Autodesk Fusion 360 part; units mm, degrees
note: some values were not read from the file. Set by a fixed rule: which sketch regions a step uses.
(part 2 of 2)
sketch "スケッチ2" plane through (0, 0, -13.6) normal (0, 0, -1) x (1, 0, 0)
  line L0 (102.5, -6.3) -> (102.5, 113.7)
  line L1 (-7.5, 113.7) -> (-7.5, -6.3)
  line L2 (-7.5, -6.3) -> (102.5, -6.3)
  line L3 (102.5, -6.3) -> (-7.5, -6.3)
  line L4 (102.5, -6.3) -> (88.1851, -6.3)
  line L5 (6.8149, -6.3) -> (-7.5, -6.3)
  arc A0 (79.5945, -2.1704) -> (15.4055, -2.1704) centre (47.5, -27.8382) ccw
  arc A1 (79.5945, -2.1704) -> (88.1851, -6.3) centre (88.1851, 4.7) ccw
  arc A2 (6.8149, -6.3) -> (15.4055, -2.1704) centre (6.8149, 4.7) ccw
  dimension "d131" = 11
  dimension "d132" = 11
  constraint coincident L0.start L2.end
  constraint coincident L1.end L2.start
  constraint tangent L4 A1
  constraint tangent A0 A1
  constraint tangent L5 A2
  constraint tangent A0 A2
  measures "d131" radius of A1
  measures "d132" radius of A2
sketch "スケッチ3" plane through (-7.5, 0, 0) normal (-1, 0, 0) x (0, -1, 0)
  line L0 (-6.3, 0) -> (-6.3, -13.6)
  line L1 (-6.3, -13.6) -> (113.7, -13.6)
  line L2 (113.7, -13.6) -> (113.7, 0)
  line L3 (113.7, -13.6) -> (-6.3, -13.6)
  line L4 (-6.3, -13.6) -> (-6.3, -26.6)
  line L5 (62.6427, -19.1312) -> (113.7, -13.6)
  line L6 (-6.3, -13.6) -> (-4.908, -26.4492)
  line L7 (113.7, -13.6) -> (112.2266, 0.0005)
  line L8 (112.2266, 0.0005) -> (113.7, 0)
  line L9 (113.7, -13.6) -> (113.7, 0)
  line L10 (113.7, 0) -> (103.9, 0)
  line L11 (103.9, 0) -> (95.0048, 0.2938)
  line L12 (103.9, 0) -> (113.7, -13.6)
  line L13 (113.7, 0) -> (113.6982, -5)
  line L14 (113.6982, -5) -> (113.6982, -8)
  line L15 (95.0048, 0.2938) -> (94.7516, -7.3743)
  line L16 (103.9, 0) -> (103.6468, -7.668)
  line L17 (113.6982, -5) -> (94.8506, -4.3775)
  line L18 (113.6982, -8) -> (94.7516, -7.3743)
  line L19 (95.0048, 0.2938) -> (107.3519, -4.7904)
  line L20 (-4.908, -26.4492) -> (113.7, -13.6)
  line L21 (15.8428, -24.2012) -> (-4.908, -26.4492)
  line L22 (24.744, -23.2369) -> (-4.908, -26.4492)
  line L23 (9.918, -24.8431) -> (9.918, -13.6)
  arc A0 (58.2791, -18.1695) -> (19.8991, -22.3273) centre (41.8256, -45.5076) ccw
  arc A1 (15.8428, -24.2012) -> (19.8991, -22.3273) centre (15.0888, -17.2419) ccw
  arc A2 (58.2791, -18.1695) -> (62.6427, -19.1312) centre (61.8888, -12.1719) ccw
  line L24 (113.7, 0) -> (125.4418, 0)
  line L25 (125.4418, 0) -> (125.4418, -18.6195)
  line L26 (125.4418, -18.6195) -> (113.7, -18.6195)
  line L27 (113.7, -18.6195) -> (113.7, 0)
  line L28 (-4.908, -26.4492) -> (-6.3, -26.6)
  line L29 (-6.3, -13.6) -> (128.5492, -13.6)
  line L30 (128.5492, -13.6) -> (128.5492, -27.0128)
  line L31 (128.5492, -27.0128) -> (-6.3, -27.0128)
  line L32 (-6.3, -27.0128) -> (-6.3, -13.6)
  line L33 (113.7, 0) -> (-6.3, 0)
  dimension "d133" = 13
  dimension "d146" = 9.8
  dimension "d147" = 8.9
  dimension "d148" = 5
  dimension "d149" = 3
  dimension "d160" = 7
  dimension "d161" = 7
  constraint coincident L1.end L2.start
  constraint coincident L0.end L1.start
  constraint perpendicular L3 L4
  constraint coincident L5 L6.end
  constraint perpendicular L5 L6
  constraint perpendicular L5 L7
  constraint coincident L2.end L8.end
  constraint perpendicular L9 L10
  constraint perpendicular L8 L13
  constraint parallel L9 L14
  constraint perpendicular L11 L15
  constraint perpendicular L11 L16
  constraint coincident L15 L17.end
  constraint perpendicular L15 L17
  constraint perpendicular L15 L18
  constraint coincident L18 L16.end
  constraint coincident L12 L19.end
  constraint coincident L17 L19.end
  constraint midpoint L22 L23.start
  constraint coincident L3 L23.end
  constraint perpendicular L3 L23
  constraint tangent L23 A0
  constraint tangent L3 A0
  constraint coincident L21 L22.start
  constraint tangent A0 A1
  constraint tangent L21 A1
  constraint tangent A0 A2
  constraint tangent L5 A2
  constraint horizontal L24
  constraint vertical L25
  constraint horizontal L26
  constraint vertical L27
  constraint parallel L22 L28
  constraint horizontal L29
  constraint vertical L30
  constraint horizontal L31
  constraint vertical L32
  measures "d133" distance of L0.end L4.end
  measures "d146" distance of L2.end L10.end
  measures "d147" distance of L10.end L11.end
  measures "d148" distance of L2.end L13.end
  measures "d149" distance of L13.end L14.end
  measures "d160" radius of A1
  measures "d161" radius of A2
extrude "押し出し9" add sketch "スケッチ3" against normal blind 110 contours L1 L3 L6 L20 L21 L22 L23 L29 | L1 L3 L20 L21 L22 L23 A0 A1 L29 | L1 L3 L5 L20 A0 A2 L29 | L20 L22 A0 A1 A2
extrude "押し出し10" cut 2 faces at (11.85, -19.9223, 0) (11.85, -19.9223, 0) along direction (0, 0, -1) blind 0.1
extrude "押し出し11" cut sketch "スケッチ2" along normal blind 16 and the other way blind 2
sketch "スケッチ8" plane through (0, 6.3, 0) normal (0, 1, 0) x (-1, 0, 0)
  line L0 (-6.8149, -11.7) -> (-6.8149, -13.6)
  line L1 (-6.8149, -13.6) -> (7.5, -13.6)
  line L2 (7.5, -13.6) -> (7.5, -0.1)
  line L3 (7.5, -0.1) -> (-102.5, -0.1)
  line L4 (-102.5, -0.1) -> (-102.5, -13.6)
  line L5 (-102.5, -13.6) -> (-88.1851, -13.6)
  line L6 (-88.1851, -13.6) -> (-88.1851, -11.7)
  line L7 (-88.1851, -11.7) -> (-97.7, -11.7)
  line L8 (-97.7, -11.7) -> (-97.7, -10.5)
  line L9 (-97.7, -10.5) -> (-87.7, -10.5)
  line L10 (-87.7, -10.5) -> (-87.7, -8.7)
  line L11 (-87.7, -8.7) -> (-97.7, -8.7)
  line L12 (-97.7, -8.7) -> (-97.7, -2.9)
  line L13 (-97.7, -2.9) -> (2.7, -2.9)
  line L14 (2.7, -2.9) -> (2.7, -8.7)
  line L15 (2.7, -8.7) -> (-7.3, -8.7)
  line L16 (-7.3, -8.7) -> (-7.3, -10.5)
  line L17 (-7.3, -10.5) -> (2.7, -10.5)
  line L18 (2.7, -10.5) -> (2.7, -11.7)
  line L19 (2.7, -11.7) -> (-6.8149, -11.7)
  line L20 (-97.7, -10.5) -> (-97.7, -11.7)
  circle A0 centre (-97.7, -10.5) radius 0.2
  circle A1 centre (-97.7, -11.7) radius 0.2
  circle A2 centre (2.7, -10.5) radius 0.2
  circle A3 centre (2.7, -11.7) radius 0.2
  dimension "d182" = 0.4
  dimension "d183" = 0.4
  dimension "d184" = 0.4
  dimension "d185" = 0.4
  constraint coincident L8.end L9.start
  constraint coincident L7.end L8.start
  constraint coincident L17.end L18.start
  constraint coincident L18.end L19.start
  measures "d182" diameter of A0
  measures "d183" diameter of A1
  measures "d184" diameter of A2
  measures "d185" diameter of A3
extrude "押し出し14" cut sketch "スケッチ8" against normal blind 105 contours L18 L19 A3 | L17 L18 A2 | L7 L8 L20 A1 | L8 L9 L20 A0 picked at (2.5674, -11.7099) picked at (2.6096, -10.4025) picked at (-97.7355, -11.8282) picked at (-97.7355, -10.3718)
fillet "フィレット7" radius 0.15 8 edges at (97.5, -46.2, -10.5) (97.7, -46.2, -10.7) (97.7, -46.2, -11.5) (97.5, -46.2, -11.7) (-2.7, -46.2, -10.7) (-2.7, -46.2, -11.5) (-2.5, -46.2, -11.7) (-2.5, -46.2, -10.5)
